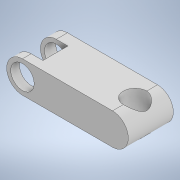
# Autodesk Inventor part: uperlegV1
Saved by Autodesk Inventor 2022 (Build 260153000, 153)
## iProperties
Created: 2022-01-23
Part Number: uperlegV1
Material: Generic
Document SubType Name: Modeling
Designer: money
Density: 1 g/cm^3
Appearance: Default
Author: money
Autodesk Inventor part; units mm, degrees
ref_plane "YZ Plane" through (0, 0, 0) normal (1, 0, 0) x (0, 1, 0)
ref_plane "XZ Plane" through (0, 0, 0) normal (0, 1, 0) x (-1, 0, 0)
ref_plane "XY Plane" through (0, 0, 0) normal (0, 0, 1) x (1, 0, 0)
sketch "Sketch1" plane through (0, 0, 0) normal (0, 0, 1) x (1, 0, 0)
  circle A0 centre (0, 0) radius 6.604
  arc A1 (0, 8.89) -> (0, -8.89) centre (0, 0) ccw
  line L0 (0, 8.89) -> (50.8, 8.89)
  arc A2 (50.8, -8.89) -> (50.8, 8.89) centre (50.8, 0) ccw
  line L1 (0, -8.89) -> (50.8, -8.89)
  dimension "d0" = 13.208
  dimension "d1" = 17.78
  dimension "d2" = 50.8
  constraints: 4 end point, 4 point on circle, 3 centre point, 2 coincident, 2 tangent, 1 horizontal
  measures "d0" diameter of A0
  measures "d1" diameter of A1
  measures "d2" distance of L0.start L0.end
extrude "Extrusion1" add sketch "Sketch1" along normal blind 25.4
sketch "Sketch2" plane through (0, 0, 0) normal (0, 1, 0) x (-1, 0, 0)
  line L0 (0, 0) -> (0, 25.4) projected
  line L1 (0, 0) -> (0, 25.4)
  line L2 (8.89, 0) -> (0, 0) projected
  line L3 (0, 0) -> (0, 12.7)
  line L4 (0, 12.7) -> (0, 25.4)
  line L5 (8.89, 0) -> (8.89, 25.4) projected
  line L6 (0, 6.35) -> (8.89, 6.35)
  line L7 (8.89, 6.35) -> (8.89, 20.4788)
  line L8 (8.89, 20.4788) -> (0, 20.4788)
  line L9 (0, 20.4788) -> (0, 6.35)
  line L10 (-6.604, 25.4) -> (-6.604, 0) projected
  line L11 (0, 6.35) -> (-6.604, 6.35)
  line L12 (-6.604, 6.35) -> (-6.604, 20.4788)
  line L13 (-6.604, 20.4788) -> (0, 20.4788)
  line L14 (0, 20.4788) -> (0, 6.35)
  constraints: 22 end point, 4 parallel, 2 collinear, 2 horizontal, 2 midpoint, 2 perpendicular, 2 point on line
extrude "Extrusion2" cut sketch "Sketch2" along normal mid plane 25.4 contours L11 L10 L13 L0 | L0 L8 L5 L6
sketch "Sketch3" plane through (0, 0, 0) normal (0, 1, 0) x (-1, 0, 0)
  line L0 (-50.8, 0) -> (-50.8, 25.4) projected
  circle A0 centre (-50.8, 12.7) radius 6.604
  point P0 (0, 0)
  dimension "d8" = 13.208
  constraints: 1 centre point, 1 midpoint
  measures "d8" diameter of A0
extrude "Extrusion3" cut sketch "Sketch3" along normal mid plane 25.4
body "Solid1"
